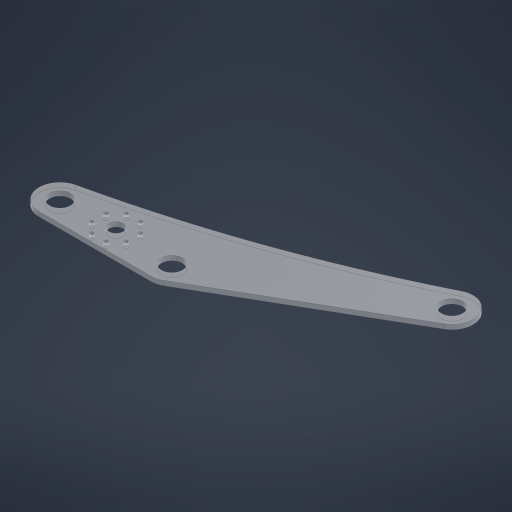
# Autodesk Inventor part: CORL_006_SmallPlate
Saved by Autodesk Inventor 2024.2 (Build 282272000, 272)
## iProperties
Created: 2024-08-02
Part Number: CORL_006_SmallPlate
Material: Polycarbonate, Clear
Document SubType Name: Modeling
Designer: Bryan
Density: 1.2 g/cm^3
Appearance: Polycarbonate - Clear
Mass: 267.729 g
Surface Area: 796.965 cm^2
Volume: 223.107 cm^3
Author: Bryan
Autodesk Inventor part; units mm, degrees
ref_plane "YZ Plane" through (0, 0, 0) normal (1, 0, 0) x (0, 1, 0)
ref_plane "XZ Plane" through (0, 0, 0) normal (0, 1, 0) x (-1, 0, 0)
ref_plane "XY Plane" through (0, 0, 0) normal (0, 0, 1) x (1, 0, 0)
sketch "Sketch1" plane through (0, 0, 0) normal (0, 1, 0) x (-1, 0, 0)
  circle A0 centre (0, 0) radius 14.2875
  line L0 (0, 0) -> (152.4, 0) construction
  circle A1 centre (152.4, 0) radius 14.2875
  circle A2 centre (0, 0) radius 28.575 construction
  circle A3 centre (152.4, 0) radius 28.575 construction
  line L1 (152.4, -28.575) -> (0, -28.575)
  line L2 (0, 28.575) -> (152.4, 28.575)
  arc A4 (152.4, -28.575) -> (152.4, 28.575) centre (152.4, 0) ccw
  arc A5 (0, 28.575) -> (0, -28.575) centre (0, 0) ccw
  dimension "d0" = 28.575
  dimension "d1" = 152.4
  dimension "d5" = 57.15
  constraints: 8 point on circle, 7 tangent, 6 centre point, 6 end point, 4 coincident, 2 equal radius, 1 horizontal
  measures "d0" diameter of A0
  measures "d1" distance of L0.start L0.end
  measures "d5" diameter of A2
extrude "Extrusion1" add sketch "Sketch1" along normal blind 6.35
sketch "Sketch3" plane through (0, 6.35, 0) normal (0, 1, 0) x (1, 0, 0)
  circle A0 centre (-152.4, 0) radius 14.2875 construction
  line L0 (0, 0) -> (-152.4, 0) construction
  circle A1 centre (0, 0) radius 14.2875 construction
  line L1 (0, 0) -> (241.9675, 139.7) construction
  arc A2 (0, -28.575) -> (0, 28.575) centre (0, 0) ccw projected
  circle A3 centre (0, 0) radius 28.575
  circle A4 centre (241.9675, 139.7) radius 28.575 construction
  circle A5 centre (241.9675, 139.7) radius 14.2875
  circle A6 centre (0, 0) radius 14.2875 projected
  line L2 (227.68, 164.4467) -> (-14.2875, 24.7467)
  line L3 (256.255, 114.9533) -> (14.2875, -24.7467)
  arc A7 (256.255, 114.9533) -> (227.68, 164.4467) centre (241.9675, 139.7) ccw
  point P0 (0, 28.575)
  point P1 (14.2875, -24.7467)
  dimension "d12" = 279.4
  dimension "d13" = 150
  constraints: 8 end point, 7 point on circle, 5 tangent, 4 centre point, 3 coincident, 2 equal radius, 1 horizontal
  measures "d12" distance of L1.start L1.end
  measures "d13" angle of L0 L1
extrude "Extrusion3" add sketch "Sketch3" against normal blind 6.35 contours A2 A3 L2 A7 L3
sketch "Sketch4" plane through (0, 6.35, 0) normal (0, 1, 0) x (1, 0, 0)
  circle A0 centre (-81.121, 5.0812) radius 30 construction
  circle A1 centre (-81.121, 5.0812) radius 25.4 construction
  circle A2 centre (-81.121, 5.0812) radius 9.6012
  circle A3 centre (0, 0) radius 40.64 construction
  circle A4 centre (-81.121, 5.0812) radius 40.64 construction
  line L0 (-90.8412, -18.3853) -> (-90.8412, 28.5478) construction
  line L1 (-90.8412, 28.5478) -> (-71.4009, 28.5478) construction
  line L2 (-71.4009, 28.5478) -> (-71.4009, -18.3853) construction
  line L3 (-71.4009, -18.3853) -> (-90.8412, -18.3853) construction
  circle A5 centre (-90.8412, -18.3853) radius 2.4892
  circle A6 centre (-71.4009, -18.3853) radius 2.4892
  circle A7 centre (-57.6545, -4.6389) radius 2.4892
  circle A8 centre (-57.6545, 14.8014) radius 2.4892
  line L4 (2.5406, 40.5605) -> (-2.5406, -40.5605) construction
  circle A9 centre (241.9675, 139.7) radius 14.2875 construction
  line L5 (-81.121, 5.0812) -> (241.9675, 139.7) construction
  circle A10 centre (241.9675, 139.7) radius 14.2875 projected
  circle A11 centre (0, 0) radius 14.2875 projected
  circle A12 centre (-152.4, 0) radius 14.2875 projected
  line L6 (-7.6566, 28.575) -> (-152.4, 28.575) projected
  arc A13 (-152.4, 28.575) -> (-152.4, -28.575) centre (-152.4, 0) ccw projected
  line L7 (-152.4, -28.575) -> (0, -28.575) projected
  arc A14 (0, -28.575) -> (14.2875, -24.7467) centre (0, 0) ccw projected
  line L8 (14.2875, -24.7467) -> (256.255, 114.9533) projected
  arc A15 (256.255, 114.9533) -> (227.68, 164.4467) centre (241.9675, 139.7) ccw projected
  line L9 (227.68, 164.4467) -> (-7.6566, 28.575) projected
  arc A16 (-152.4, 28.575) -> (-152.4, -28.575) centre (-152.4, 0) ccw projected
  circle A17 centre (0, 0) radius 50.8 construction
  arc A18 (-152.4, 28.575) -> (-152.4, -28.575) centre (-152.4, 0) ccw projected
  arc A19 (256.255, 114.9533) -> (227.68, 164.4467) centre (241.9675, 139.7) ccw projected
  line L10 (-161.9414, 26.935) -> (232.4261, 166.635)
  circle A20 centre (-71.4009, 28.5478) radius 2.4892
  circle A21 centre (-90.8412, 28.5478) radius 2.4892
  circle A22 centre (-104.5876, 14.8014) radius 2.4892
  circle A23 centre (-104.5876, -4.6389) radius 2.4892
  arc A24 (-158.6567, 27.8816) -> (229.2779, 165.3028) centre (-535.9643, 1709.2783) ccw
  point P0 (34.7284, 53.046)
  point P1 (38.9386, 55.4768)
  point P2 (-93.3302, 28.575)
  point P3 (-88.3521, 28.575)
  point P4 (-73.8899, 28.575)
  point P5 (-68.9118, 28.575)
  point P6 (229.2779, 165.3028)
  point P7 (-158.6567, 27.8816)
  dimension "d16" = 60
  dimension "d17" = 50.8
  dimension "d18" = 19.2024
  dimension "d19" = 81.28
  dimension "d21" = 4.9784
  dimension "d24" = 360
  dimension "d26" = 350.012
  dimension "d31" = 101.6
  constraints: 15 centre point, 14 end point, 11 point on circle, 9 coincident, 6 tangent, 3 parallel, 1 equal radius, 1 perpendicular, 23 other
  measures "d16" diameter of A0
  measures "d17" diameter of A1
  measures "d18" diameter of A2
  measures "d19" diameter of A3
  measures "d21" diameter of A5
  measures "d26" distance of L5.start L5.end
  measures "d31" diameter of A17
extrude "Extrusion6" add sketch "Sketch4" against normal blind 6.35 contours L6 A20 A21 A13 A24 A15 L9
extrude "Extrusion7" cut sketch "Sketch4" against normal blind 6.35 contours A2 | A5 | A6 | A7 | A8 | A20 L6 | A21 L6 | A22 | A23 picked at (-70.6668, 28.1731) picked at (-90.1071, 28.1731)
body "Solid1"
